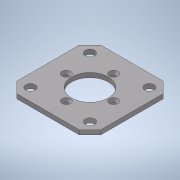
# Autodesk Inventor part: MotorMountingPlate_Draft02
Saved by Autodesk Inventor 2022 (Build 260153000, 153)
## iProperties
Created: 2021-05-22
Part Number: MotorMountingPlate_Draft02
Material: Aluminum 6061
Document SubType Name: Modeling
Designer: M3rob
Density: 2.7 g/cm^3
Appearance: Aluminum - Polished
Mass: 77.523 g
Surface Area: 150.277 cm^2
Volume: 28.7122 cm^3
Author: M3rob
Autodesk Inventor part; units mm, degrees
ref_plane "YZ Plane" through (0, 0, 0) normal (1, 0, 0) x (0, 1, 0)
ref_plane "XZ Plane" through (0, 0, 0) normal (0, 1, 0) x (-1, 0, 0)
ref_plane "XY Plane" through (0, 0, 0) normal (0, 0, 1) x (1, 0, 0)
sketch "Sketch1" plane through (0, 0, 0) normal (0, 1, 0) x (-1, 0, 0)
  line L0 (44.45, -44.45) -> (33.02, -44.45) construction
  line L1 (-44.45, -44.45) -> (-44.45, -33.02) construction
  line L2 (-44.45, 44.45) -> (-33.02, 44.45) construction
  line L3 (44.45, 44.45) -> (44.45, 33.02) construction
  line L4 (33.02, -44.45) -> (44.45, -33.02)
  line L5 (-33.02, -44.45) -> (-44.45, -33.02)
  line L6 (-44.45, 33.02) -> (-33.02, 44.45)
  line L7 (33.02, 44.45) -> (44.45, 33.02)
  line L8 (-38.735, -38.735) -> (38.735, 38.735) construction
  line L9 (38.735, -38.735) -> (-38.735, 38.735) construction
  line L10 (33.02, -44.45) -> (-33.02, -44.45)
  line L11 (44.45, -33.02) -> (44.45, -44.45) construction
  line L12 (44.45, 33.02) -> (44.45, -33.02)
  line L13 (33.02, 44.45) -> (44.45, 44.45) construction
  line L14 (-33.02, 44.45) -> (33.02, 44.45)
  line L15 (-44.45, 33.02) -> (-44.45, 44.45) construction
  line L16 (-44.45, -33.02) -> (-44.45, 33.02)
  line L17 (-33.02, -44.45) -> (-44.45, -44.45) construction
  circle A0 centre (0, 0) radius 19.3675
  circle A1 centre (0, -25.019) radius 2.3813 construction
  circle A2 centre (-31.4309, -31.4309) radius 4.7625 construction
  circle A3 centre (25.019, 0) radius 2.3813 construction
  circle A4 centre (0, 25.019) radius 2.3813 construction
  circle A5 centre (-25.019, 0) radius 2.3813 construction
  circle A6 centre (31.4309, -31.4309) radius 4.7625 construction
  circle A7 centre (31.4309, 31.4309) radius 4.7625 construction
  circle A8 centre (-31.4309, 31.4309) radius 4.7625 construction
  circle A9 centre (0, 0) radius 34.925 construction
  point P0 (44.45, 0)
  dimension "d0" = 88.9
  dimension "d1" = 11.43
  dimension "d2" = 45
  dimension "d3" = 38.735
  dimension "d6" = 360
  dimension "d10" = 360
  dimension "d12" = 25.019
  dimension "d13" = 44.45
  dimension "d14" = 9.525
  dimension "d15" = 4.7625
  dimension "d16" = 69.85
  constraints: 36 end point, 18 parallel, 14 perpendicular, 10 centre point, 6 midpoint, 3 coincident, 3 horizontal, 2 point on line, 1 horizontal alignment, 1 vertical alignment, 18 other
  measures "d0" distance of L1.start L2.start
  measures "d1" distance of L0.end L0.start
  measures "d2" angle of L10 L9
  measures "d3" diameter of A0
  measures "d12" distance of point (0, 0) A1.centre
  measures "d13" distance of point (0, 0) A6.centre
  measures "d14" diameter of A7
  measures "d15" diameter of A4
  measures "d16" diameter of A9
extrude "Extrusion1" add sketch "Sketch1" against normal blind 4.7625
sketch "Sketch2" plane through (0, 0, 0) normal (0, 1, 0) x (1, 0, 0)
  circle A0 centre (0, 0) radius 44.45 construction
  point P0 (-31.4309, -31.4309)
  point P1 (-31.4309, 31.4309)
  point P2 (31.4309, 31.4309)
  point P3 (31.4309, -31.4309)
  point P4 (25.019, 0)
  point P5 (0, -25.019)
  point P6 (-25.019, 0)
  point P7 (0, 25.019)
  constraints: 1 coincident, 3 other
hole "Hole1" at (25.019, 0, 0) at (0, 0, 25.019) at (-25.019, 0, 0) at (0, 0, -25.019) direction (0, -1, 0) diameter 4.4958 end through all countersink diameter 9.144 countersink angle 82 clearance for "Flat Head Machine Screw (82)" size "#8" standard "Ansi Unified Screw Threads"
hole "Hole2" at (-31.4309, 0, 31.4309) at (-31.4309, 0, -31.4309) at (31.4309, 0, -31.4309) at (31.4309, 0, 31.4309) direction (0, -1, 0) diameter 10.0838 end through all clearance for "Flat Head Machine Screw (82)" size "3/8" standard "Ansi Unified Screw Threads"
body "Solid1"
